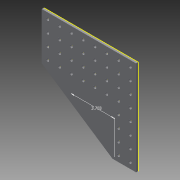
# Autodesk Inventor part: 2020-2040_mounting_plate
Saved by Autodesk Inventor 2014 (Build 180170000, 170)
## iProperties
Created: 2014-09-28
Part Number: 2020-2040_mounting_plate
Material: Generic
Document SubType Name: Modeling
Designer: Matthew
Density: 1 g/cm^3
Appearance: Default
Author: Matthew
Autodesk Inventor part; units mm, degrees
ref_plane "YZ Plane" through (0, 0, 0) normal (1, 0, 0) x (0, 1, 0)
ref_plane "XZ Plane" through (0, 0, 0) normal (0, 1, 0) x (-1, 0, 0)
ref_plane "XY Plane" through (0, 0, 0) normal (0, 0, 1) x (1, 0, 0)
sketch "Sketch1" plane through (0, 0, 0) normal (0, 0, 1) x (1, 0, 0)
  line L0 (-136.0714, 83.0036) -> (16.3286, -18.5964)
  line L1 (16.3286, -18.5964) -> (67.1286, -18.5964)
  line L2 (67.1286, -18.5964) -> (67.1286, 184.6036)
  line L3 (67.1286, 184.6036) -> (-136.0714, 184.6036)
  line L4 (-136.0714, 184.6036) -> (-136.0714, 83.0036)
  point P0 (0, 0)
  dimension "d0" = 101.6
  dimension "d1" = 50.8
  dimension "d2" = 203.2
  dimension "d4" = 203.2
  constraints: 10 end point, 1 parallel, 1 perpendicular
  measures "d0" distance of L3.end L0.start
  measures "d1" distance of L0.end L1.end
  measures "d2" distance of L1.end L2.end
  measures "d4" distance of L2.end L3.end
extrude "Extrusion1" add sketch "Sketch1" along normal blind 4.7625
sketch "Sketch2" plane through (0, 0, 4.7625) normal (0, 0, 1) x (1, 0, 0)
  line L0 (16.3286, -18.5964) -> (67.1286, -18.5964) projected
  line L1 (67.1286, -18.5964) -> (67.1286, 184.6036) projected
  line L2 (67.1286, 184.6036) -> (-136.0714, 184.6036) projected
  line L3 (-136.0714, 184.6036) -> (-136.0714, 83.0036) projected
  point P0 (0, 0)
  point P1 (-123.3714, 171.9036)
  point P2 (-97.9714, 171.9036)
  point P3 (-72.5714, 171.9036)
  point P4 (-47.1714, 171.9036)
  point P5 (-21.7714, 171.9036)
  point P6 (3.6286, 171.9036)
  point P7 (29.0286, 171.9036)
  point P8 (54.4286, 171.9036)
  point P9 (-123.3714, 146.5036)
  point P10 (-97.9714, 146.5036)
  point P11 (-72.5714, 146.5036)
  point P12 (-47.1714, 146.5036)
  point P13 (-21.7714, 146.5036)
  point P14 (3.6286, 146.5036)
  point P15 (29.0286, 146.5036)
  point P16 (54.4286, 146.5036)
  point P17 (-123.3714, 121.1036)
  point P18 (-97.9714, 121.1036)
  point P19 (-72.5714, 121.1036)
  point P20 (-47.1714, 121.1036)
  point P21 (-21.7714, 121.1036)
  point P22 (3.6286, 121.1036)
  point P23 (29.0286, 121.1036)
  point P24 (54.4286, 121.1036)
  point P25 (-123.3714, 95.7036)
  point P26 (-97.9714, 95.7036)
  point P27 (-72.5714, 95.7036)
  point P28 (-47.1714, 95.7036)
  point P29 (-21.7714, 95.7036)
  point P30 (3.6286, 95.7036)
  point P31 (29.0286, 95.7036)
  point P32 (54.4286, 95.7036)
  point P33 (54.4286, 70.3036)
  point P34 (54.4286, 44.9036)
  point P35 (54.4286, 19.5036)
  point P36 (54.4286, -5.8964)
  point P37 (29.0286, 95.7036)
  point P38 (29.0286, 70.3036)
  point P39 (29.0286, 44.9036)
  point P40 (29.0286, 19.5036)
  point P41 (29.0286, -5.8964)
  dimension "d26" = 12.7
  dimension "d27" = 12.7
  dimension "d30" = 25.4
  dimension "d33" = 25.4
  dimension "d38" = 25.4
  dimension "d41" = 25.4
  constraints: 2 horizontal, 2 vertical, 40 other
  measures "d26" distance from line of L3 point (-123.371, 171.904)
  measures "d27" distance from line of L2 point (-123.371, 171.904)
  measures "d30" distance of point (-123.371, 171.904) point (-97.971, 171.904)
  measures "d33" distance of point (-123.371, 171.904) point (-123.371, 146.504)
  measures "d38" distance of point (54.429, 95.704) point (54.429, 70.304)
  measures "d41" distance of point (54.429, 95.704) point (29.029, 95.704)
hole "Hole1" at (-123.3714, 171.9036, 4.7625) at (-97.9714, 171.9036, 4.7625) at (-72.5714, 171.9036, 4.7625) at (-47.1714, 171.9036, 4.7625) at (-21.7714, 171.9036, 4.7625) at (3.6286, 171.9036, 4.7625) at (29.0286, 171.9036, 4.7625) at (54.4286, 171.9036, 4.7625) at (-123.3714, 146.5036, 4.7625) at (-97.9714, 146.5036, 4.7625) at (-72.5714, 146.5036, 4.7625) at (-47.1714, 146.5036, 4.7625) at (-21.7714, 146.5036, 4.7625) at (3.6286, 146.5036, 4.7625) at (29.0286, 146.5036, 4.7625) at (54.4286, 146.5036, 4.7625) at (-123.3714, 121.1036, 4.7625) at (-97.9714, 121.1036, 4.7625) at (-72.5714, 121.1036, 4.7625) at (-47.1714, 121.1036, 4.7625) at (-21.7714, 121.1036, 4.7625) at (3.6286, 121.1036, 4.7625) at (29.0286, 121.1036, 4.7625) at (54.4286, 121.1036, 4.7625) at (-123.3714, 95.7036, 4.7625) at (-97.9714, 95.7036, 4.7625) at (-72.5714, 95.7036, 4.7625) at (-47.1714, 95.7036, 4.7625) at (-21.7714, 95.7036, 4.7625) at (3.6286, 95.7036, 4.7625) at (29.0286, 95.7036, 4.7625) at (54.4286, 95.7036, 4.7625) at (54.4286, 70.3036, 4.7625) at (54.4286, 44.9036, 4.7625) at (54.4286, 19.5036, 4.7625) at (54.4286, -5.8964, 4.7625) at (29.0286, 70.3036, 4.7625) at (29.0286, 44.9036, 4.7625) at (29.0286, 19.5036, 4.7625) at (29.0286, -5.8964, 4.7625) direction (0, 0, -1) diameter 6.35 end through all
sketch "Sketch3" plane through (0, 0, 0) normal (0, 0, -1) x (-1, 0, 0)
  line L0 (136.0714, 83.0036) -> (-16.3286, -18.5964) projected
  line L1 (33.684, 65.5453) -> (109.884, 65.5453)
  line L2 (33.684, 65.5453) -> (33.684, 14.7453)
  point P0 (0, 0)
  dimension "d53" = 50.8
  dimension "d54" = 33.3417
  dimension "d55" = 76.2
  constraints: 4 end point, 2 point on line, 1 perpendicular
  measures "d53" distance of L1.start L2.end
  measures "d54" vertical distance of L0.end L2.end
  measures "d55" distance of L1.start L1.end
extrude "Extrusion2" cut sketch "Sketch3" against normal blind 25.4
equation "\"d4\" = d2"
body "Solid1"
